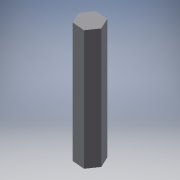
# Autodesk Inventor part: Hex Shaft
Saved by Autodesk Inventor 2017 (Build 210142000, 142)
## iProperties
Created: 2017-12-29
Part Number: Hex Shaft
Material: Generic
Document SubType Name: Modeling
Designer: anikasoojin
Density: 1 g/cm^3
Appearance: Default
Author: anikasoojin
Autodesk Inventor part; units mm, degrees
ref_plane "YZ Plane" through (0, 0, 0) normal (1, 0, 0) x (0, 1, 0)
ref_plane "XZ Plane" through (0, 0, 0) normal (0, 1, 0) x (-1, 0, 0)
ref_plane "XY Plane" through (0, 0, 0) normal (0, 0, 1) x (1, 0, 0)
sketch "Sketch1" plane through (0, 0, 0) normal (0, 1, 0) x (-1, 0, 0)
  line L0 (-8.2612, 21.3942) -> (-12.4421, 15.3706)
  line L1 (-12.4421, 15.3706) -> (-19.7491, 15.9795)
  line L2 (-19.7491, 15.9795) -> (-22.8753, 22.612)
  line L3 (-22.8753, 22.612) -> (-18.6944, 28.6356)
  line L4 (-18.6944, 28.6356) -> (-11.3874, 28.0267)
  line L5 (-11.3874, 28.0267) -> (-8.2612, 21.3942)
  point P0 (0, 0)
  point P1 (-15.5682, 22.0031)
  dimension "d0" = 12.7
  constraints: 12 end point, 13 other
  measures "d0" distance between parallel lines of L1 L4
extrude "Extrusion1" add sketch "Sketch1" along normal blind 58.42
sketch "Sketch4" plane through (0, 58.42, 0) normal (0, 1, 0) x (1, 0, 0)
  circle A0 centre (16.0831, -22.124) radius 3.175
  point P0 (0, 0)
  dimension "d4" = 6.35
  constraints: 1 centre point
  measures "d4" diameter of A0
extrude "Extrusion2" cut sketch "Sketch4" against normal through all
body "Solid1"
